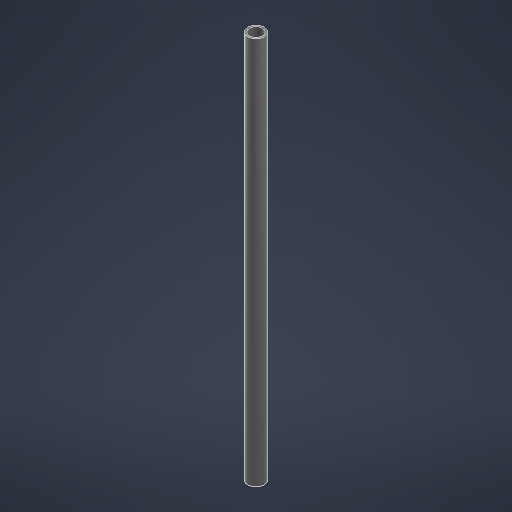
# Autodesk Inventor part: Carbonrohr
Saved by Autodesk Inventor 2025.2 (Build 292293000, 293)
## iProperties
Created: 2024-11-26
Part Number: Carbonrohr
Material: Generisch
Document SubType Name: Modeling
Designer: Fabian
Density: 1 g/cm^3
Appearance: Glatt - Schwarz
Author: Fabian
Autodesk Inventor part; units mm, degrees
ref_plane "YZ Plane" through (0, 0, 0) normal (1, 0, 0) x (0, 1, 0)
ref_plane "XZ Plane" through (0, 0, 0) normal (0, 1, 0) x (-1, 0, 0)
ref_plane "XY Plane" through (0, 0, 0) normal (0, 0, 1) x (1, 0, 0)
sketch "Skizze1" plane through (0, 0, 0) normal (0, 1, 0) x (-1, 0, 0)
  circle A0 centre (0, 0) radius 2
  circle A1 centre (0, 0) radius 2.5
  dimension "d0" = 4
  dimension "d1" = 0.5
  constraints: 2 centre point, 2 coincident
  measures "d0" diameter of A0
  measures "d1" radial gap between concentric circles of A0 A1
extrude "Extrusion1" add sketch "Skizze1" along normal blind 117
